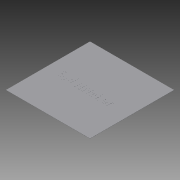
# Autodesk Inventor part: test
Saved by Autodesk Inventor 2015 SP1 (Build 190203100, 203)
## iProperties
Created: 2015-01-20
Part Number: test
Material: Generic
Document SubType Name: Modeling
Designer: Patrick
Density: 1 g/cm^3
Appearance: Default
Author: Patrick
Autodesk Inventor part; units mm, degrees
ref_plane "YZ Plane" through (0, 0, 0) normal (1, 0, 0) x (0, 1, 0)
ref_plane "XZ Plane" through (0, 0, 0) normal (0, 1, 0) x (-1, 0, 0)
ref_plane "XY Plane" through (0, 0, 0) normal (0, 0, 1) x (1, 0, 0)
sketch "Sketch1" plane through (0, 0, 0) normal (0, 0, 1) x (1, 0, 0)
  line L0 (-2500, 2500) -> (2500, 2500)
  line L1 (2500, 2500) -> (2500, -2500)
  line L2 (2500, -2500) -> (-2500, -2500)
  line L3 (-2500, -2500) -> (-2500, 2500)
  line L4 (-2500, 2500) -> (2500, -2500) construction
  line L5 (2500, 2500) -> (-2500, -2500) construction
  point P0 (0, 0)
  dimension "d0" = 5000
  dimension "d1" = 5000
  constraints: 12 end point, 2 midpoint, 2 parallel, 1 horizontal, 1 perpendicular
  measures "d0" distance of L1.end L2.end
  measures "d1" distance of L0.end L1.end
extrude "Extrusion1" add sketch "Sketch1" along normal blind 10
sketch "Sketch2" plane through (0, 0, 10) normal (0, 0, 1) x (1, 0, 0)
  spline S0 degree 4 poles (-1762.1962, 1575.4295) (-1491.5954, 1596.7242) (-1645.2682, 1599.4427) (-955.1929, 1604.26) (-825.0031, 1592.0214) (-732.519, 1582.853) (-459.1878, 1545.7413) (-345.6079, 1530.4798) (-181.1613, 1505.3471) (-45.0314, 1482.7736) (33.2926, 1462.2915) (239.3471, 1405.6013) (464.1859, 1340.1213) (686.0681, 1238.9414) (872.8585, 1134.1355) (1059.3908, 984.8503) (1135.6727, 916.3268) (1228.891, 830.1566) (1303.68, 755.6016) (1398.7078, 654.9396) (1484.4134, 536.3515) (1554.6482, 423.2358) (1622.964, 278.6899) (1656.5725, 195.5181) (1688.0679, 109.6167) (1711.1354, 34.6912) (1726.7352, -56.2271) (1732.0908, -96.9036) (1745.8175, -221.0892) (1754.6807, -282.6204) (1757.8584, -312.0265) (1759.1649, -327.9955) (1751.7151, -450.1044) (1749.3478, -483.8897) (1742.4101, -550.3074) (1733.7713, -624.2147) (1724.9155, -692.4119) (1713.0594, -760.8257) (1693.9812, -834.1715) (1666.2811, -923.9302) (1643.7916, -992.4869) (1601.981, -1107.4142) (1598.9852, -1125.3949) (1552.4445, -1217.5749) (1546.4569, -1240.9001) (1522.3305, -1296.4362) (1488.9966, -1328.7325) (1439.4405, -1364.0425) (1390.8946, -1389.0179) (1235.7237, -1476.0426) (1078.0613, -1526.58) (1029.0921, -1562.0631) (774.2297, -1615.128) (793.6908, -1622.9048) (755.7069, -1618.0314) (746.9426, -1630.276) (794.5654, -1458.788) (838.2853, -1308.0396) (850.1486, -1200.7586) (788.6595, -1247.2043) (738.5107, -1232.948) (505.6315, -1319.0728) (371.9051, -1351.4552) (170.8434, -1425.6846) (0.3667, -1497.8904) (-158.3591, -1567.0933) (-305.4965, -1632.8743) (-464.732, -1704.8026) (-562.0019, -1750.703) (-667.0386, -1801.7065) (-771.6429, -1855.0863) (-855.1097, -1895.1947) (-942.1183, -1946.1312) (-1006.5826, -1969.258) (-1131.0376, -2063.8301) (-1044.5072, -1892.2007) (-1066.3114, -1908.4549) (-1003.7573, -1699.41) (-977.9555, -1570.6674) (-934.5888, -1396.7403) (-900.0619, -1241.8358) (-878.6191, -1126.4711) (-860.2727, -1014.4476) (-841.1424, -887.8249) (-829.3125, -810.2865) (-819.1465, -727.3894) (-810.8924, -648.5496) (-803.9347, -562.191) (-795.8323, -453.4885) (-789.5667, -352.3094) (-784.6857, -245.5127) (-781.7139, -146.1831) (-779.9272, -44.8844) (-781.2254, 55.4386) (-787.9793, 179.1486) (-811.3684, 376.6004) (-842.439, 538.5854) (-892.2084, 725.6609) (-936.4315, 857.2935) (-978.7899, 950.9207) (-1037.4119, 1054.4206) (-1088.0468, 1135.0533) (-1275.6307, 1378.281) (-1438.3377, 1466.0297) (-1614.8909, 1557.3421) (-1762.1962, 1575.4295) knots 0 0 0 0 0 0.034839 0.046927 0.059157 0.069708 0.081008 0.092632 0.102748 0.113022 0.124139 0.136453 0.150242 0.164315 0.177048 0.188474 0.198679 0.20821 0.218183 0.228603 0.239498 0.249955 0.2597 0.268704 0.276906 0.284701 0.293012 0.300958 0.30789 0.314001 0.319872 0.325799 0.332476 0.340159 0.347396 0.354762 0.362372 0.370178 0.378285 0.38679 0.394808 0.402697 0.409774 0.416193 0.422676 0.428714 0.435047 0.442657 0.451726 0.462242 0.473798 0.483006 0.490066 0.494813 0.499083 0.50655 0.514493 0.522901 0.530604 0.537808 0.54693 0.558108 0.570873 0.583364 0.595556 0.607419 0.618543 0.629115 0.639153 0.64851 0.657648 0.666651 0.67507 0.683395 0.690966 0.698954 0.708235 0.71845 0.730094 0.741477 0.752176 0.762313 0.771652 0.780544 0.78896 0.796972 0.80531 0.814025 0.823107 0.832341 0.841416 0.850322 0.859373 0.869335 0.880255 0.892159 0.904186 0.91528 0.925458 0.934737 0.944559 0.95535 0.967093 1 1 1 1 1
  spline S1 degree 3 poles (809.627, -1569.6922) (882.146, -1551.6939) (955.9648, -1539.7281) (1025.1004, -1514.7845) (1138.5967, -1473.8468) (1251.7259, -1429.4464) (1342.7492, -1345.1899) (1381.8811, -1308.975) (1386.3757, -1249.1759) (1322.7566, -1223.4286) (1264.9716, -1200.0626) (1228.2905, -1195.0521) (1143.7263, -1201.3922) (1059.1523, -1207.7322) (987.8338, -1206.8988) (893.0005, -1228.9154) (866.6877, -1326.5963) (832.7748, -1465.8498) (809.627, -1569.6922) knots 0 0 0 0 1 1 1 2 2 2 3 3 3 4 4 4 5 5 5 6 6 6 6
  line L0 (-1821.1799, -36.4172) -> (-1734.2301, -27.9919)
  spline S2 degree 2 poles (-1734.2301, -27.9919) (-1726.4787, -71.8038) (-1678.2856, -112.9195) (-1637.8439, -112.9195) knots 0 0 0 1 2 2 2
  spline S3 degree 2 poles (-1637.8439, -112.9195) (-1594.706, -112.9195) (-1550.8941, -76.522) (-1550.8941, -51.9199) knots 0 0 0 1 2 2 2
  spline S4 degree 2 poles (-1550.8941, -51.9199) (-1550.8941, -36.0802) (-1569.4299, -14.1743) (-1592.3469, -6.0859) knots 0 0 0 1 2 2 2
  spline S5 degree 2 poles (-1592.3469, -6.0859) (-1607.8496, -0.6937) (-1663.794, 13.1239) knots 0 0 0 1 1 1
  spline S6 degree 2 poles (-1663.794, 13.1239) (-1735.5781, 30.9857) (-1764.5614, 56.9358) knots 0 0 0 1 1 1
  spline S7 degree 2 poles (-1764.5614, 56.9358) (-1805.3402, 93.3334) (-1805.3402, 145.5707) knots 0 0 0 1 1 1
  spline S8 degree 2 poles (-1805.3402, 145.5707) (-1805.3402, 179.6092) (-1766.9205, 238.2497) (-1694.7994, 268.918) (-1643.9102, 268.918) knots 0 0 0 1 2 3 3 3
  spline S9 degree 2 poles (-1643.9102, 268.918) (-1560.6675, 268.918) (-1476.4139, 196.1229) (-1474.3918, 135.1232) knots 0 0 0 1 2 2 2
  line L1 (-1474.3918, 135.1232) -> (-1563.7007, 131.079)
  spline S10 degree 2 poles (-1563.7007, 131.079) (-1569.4299, 165.1175) (-1607.1756, 195.1118) (-1644.9212, 195.1118) knots 0 0 0 1 2 2 2
  spline S11 degree 2 poles (-1644.9212, 195.1118) (-1684.0149, 195.1118) (-1705.9208, 179.2721) knots 0 0 0 1 1 1
  spline S12 degree 2 poles (-1705.9208, 179.2721) (-1720.0755, 168.8247) (-1720.0755, 151.6369) knots 0 0 0 1 1 1
  spline S13 degree 2 poles (-1720.0755, 151.6369) (-1720.0755, 136.1343) (-1706.9319, 124.6758) knots 0 0 0 1 1 1
  spline S14 degree 2 poles (-1706.9319, 124.6758) (-1689.7441, 110.5212) (-1559.3195, 79.8528) (-1496.9718, 47.1624) (-1461.5852, -9.7931) (-1461.5852, -51.9199) knots 0 0 0 1 2 3 4 4 4
  spline S15 degree 2 poles (-1461.5852, -51.9199) (-1461.5852, -89.6655) (-1503.7121, -156.0574) (-1580.8884, -188.4108) (-1638.5179, -188.4108) knots 0 0 0 1 2 3 3 3
  spline S16 degree 2 poles (-1638.5179, -188.4108) (-1722.4346, -188.4108) (-1812.4175, -110.8975) (-1821.1799, -36.4172) knots 0 0 0 1 2 2 2
  line L2 (-1389.4641, 139.8414) -> (-1310.2657, 139.8414)
  line L3 (-1310.2657, 139.8414) -> (-1310.2657, 92.6594)
  spline S17 degree 2 poles (-1310.2657, 92.6594) (-1294.763, 116.9244) (-1242.5257, 146.9187) (-1210.5093, 146.9187) knots 0 0 0 1 2 2 2
  spline S18 degree 2 poles (-1210.5093, 146.9187) (-1154.5649, 146.9187) (-1076.7145, 59.6319) (-1076.7145, -18.5555) knots 0 0 0 1 2 2 2
  spline S19 degree 2 poles (-1076.7145, -18.5555) (-1076.7145, -98.7649) (-1155.2389, -187.7368) (-1210.8463, -187.7368) knots 0 0 0 1 2 2 2
  spline S20 degree 2 poles (-1210.8463, -187.7368) (-1237.4705, -187.7368) (-1280.6084, -166.5049) (-1304.5364, -140.8918) knots 0 0 0 1 2 2 2
  line L4 (-1304.5364, -140.8918) -> (-1304.5364, -302.6588)
  line L5 (-1304.5364, -302.6588) -> (-1389.4641, -302.6588)
  line L6 (-1389.4641, -302.6588) -> (-1389.4641, 139.8414)
  spline S21 degree 2 poles (-1305.8845, -14.8483) (-1305.8845, -68.7706) (-1262.7466, -120.3339) (-1232.0783, -120.3339) knots 0 0 0 1 2 2 2
  spline S22 degree 2 poles (-1232.0783, -120.3339) (-1202.421, -120.3339) (-1162.9903, -73.1518) (-1162.9903, -19.2295) knots 0 0 0 1 2 2 2
  spline S23 degree 2 poles (-1162.9903, -19.2295) (-1162.9903, 30.9857) (-1203.432, 79.8528) (-1233.4263, 79.8528) knots 0 0 0 1 2 2 2
  spline S24 degree 2 poles (-1233.4263, 79.8528) (-1264.7687, 79.8528) (-1305.8845, 31.9967) (-1305.8845, -14.8483) knots 0 0 0 1 2 2 2
  line L7 (-1009.3116, -180.6595) -> (-1009.3116, 139.8414)
  line L8 (-1009.3116, 139.8414) -> (-924.3839, 139.8414)
  line L9 (-924.3839, 139.8414) -> (-924.3839, -180.6595)
  line L10 (-924.3839, -180.6595) -> (-1009.3116, -180.6595)
  line L11 (-1009.3116, 182.9793) -> (-1009.3116, 261.5037)
  line L12 (-1009.3116, 261.5037) -> (-924.3839, 261.5037)
  line L13 (-924.3839, 261.5037) -> (-924.3839, 182.9793)
  line L14 (-924.3839, 182.9793) -> (-1009.3116, 182.9793)
  line L15 (-690.1488, -295.5815) -> (-690.1488, 146.5817)
  line L16 (-690.1488, 146.5817) -> (-603.5361, 146.5817)
  line L17 (-603.5361, 146.5817) -> (-421.8852, -149.9912)
  line L18 (-421.8852, -149.9912) -> (-421.8852, 146.5817)
  line L19 (-421.8852, 146.5817) -> (-339.3166, 146.5817)
  line L20 (-339.3166, 146.5817) -> (-339.3166, -295.5815)
  line L21 (-339.3166, -295.5815) -> (-428.6255, -295.5815)
  line L22 (-428.6255, -295.5815) -> (-607.5802, -5.4119)
  line L23 (-607.5802, -5.4119) -> (-607.5802, -295.5815)
  line L24 (-607.5802, -295.5815) -> (-690.1488, -295.5815)
  line L25 (-243.9415, -295.5815) -> (-243.9415, 146.5817)
  line L26 (-243.9415, 146.5817) -> (-157.3287, 146.5817)
  line L27 (-157.3287, 146.5817) -> (24.3222, -149.9912)
  line L28 (24.3222, -149.9912) -> (24.3222, 146.5817)
  line L29 (24.3222, 146.5817) -> (106.8908, 146.5817)
  line L30 (106.8908, 146.5817) -> (106.8908, -295.5815)
  line L31 (106.8908, -295.5815) -> (17.5819, -295.5815)
  line L32 (17.5819, -295.5815) -> (-161.3729, -5.4119)
  line L33 (-161.3729, -5.4119) -> (-161.3729, -295.5815)
  line L34 (-161.3729, -295.5815) -> (-243.9415, -295.5815)
  line L35 (263.9396, -72.8148) -> (187.1003, -58.9972)
  spline S25 degree 2 poles (187.1003, -58.9972) (200.2438, -12.4892) (263.6026, 31.9967) (325.9503, 31.9967) knots 0 0 0 1 2 2 2
  spline S26 degree 2 poles (325.9503, 31.9967) (382.9058, 31.9967) (438.5132, 5.0356) (461.0932, -36.0802) (461.0932, -91.3506) knots 0 0 0 1 2 3 3 3
  line L36 (461.0932, -91.3506) -> (459.7451, -190.4329)
  spline S27 degree 2 poles (459.7451, -190.4329) (459.7451, -232.5597) (467.8335, -272.6645) (478.9549, -295.5815) knots 0 0 0 1 2 2 2
  line L37 (478.9549, -295.5815) -> (395.0383, -295.5815)
  spline S28 degree 2 poles (395.0383, -295.5815) (391.6682, -287.1561) (386.9499, -270.6424) knots 0 0 0 1 1 1
  spline S29 degree 2 poles (386.9499, -270.6424) (384.9279, -262.8911) (383.9168, -260.532) knots 0 0 0 1 1 1
  spline S30 degree 2 poles (383.9168, -260.532) (362.3479, -281.4269) (312.8067, -302.6588) (284.8345, -302.6588) knots 0 0 0 1 2 2 2
  spline S31 degree 2 poles (284.8345, -302.6588) (235.2934, -302.6588) (178.3379, -249.0735) (178.3379, -207.9577) knots 0 0 0 1 2 2 2
  spline S32 degree 2 poles (178.3379, -207.9577) (178.3379, -180.6595) (204.288, -138.1957) (251.133, -115.6157) (295.282, -107.1903) knots 0 0 0 1 2 3 3 3
  spline S33 degree 2 poles (295.282, -107.1903) (354.5965, -96.0688) (377.5135, -86.2954) knots 0 0 0 1 1 1
  line L38 (377.5135, -86.2954) -> (377.5135, -77.87)
  spline S34 degree 2 poles (377.5135, -77.87) (377.5135, -53.605) (353.2485, -32.7101) (319.884, -32.7101) knots 0 0 0 1 2 2 2
  spline S35 degree 2 poles (319.884, -32.7101) (297.3041, -32.7101) (271.6909, -50.5718) (263.9396, -72.8148) knots 0 0 0 1 2 2 2
  spline S36 degree 2 poles (377.5135, -141.5658) (361.3368, -146.958) (290.5638, -162.1237) (279.7793, -169.201) knots 0 0 0 1 2 2 2
  spline S37 degree 2 poles (279.7793, -169.201) (263.2656, -180.9965) (263.2656, -199.1953) knots 0 0 0 1 1 1
  spline S38 degree 2 poles (263.2656, -199.1953) (263.2656, -217.0571) (289.8897, -243.0072) (310.4476, -243.0072) knots 0 0 0 1 2 2 2
  spline S39 degree 2 poles (310.4476, -243.0072) (333.3646, -243.0072) (353.9225, -227.8415) knots 0 0 0 1 1 1
  spline S40 degree 2 poles (353.9225, -227.8415) (369.4252, -216.383) (374.1434, -199.8693) knots 0 0 0 1 1 1
  spline S41 degree 2 poles (374.1434, -199.8693) (377.5135, -189.0849) (377.5135, -158.4165) knots 0 0 0 1 1 1
  line L39 (377.5135, -158.4165) -> (377.5135, -141.5658)
  line L40 (541.3026, -295.5815) -> (541.3026, 146.5817)
  line L41 (541.3026, 146.5817) -> (626.2303, 146.5817)
  line L42 (626.2303, 146.5817) -> (626.2303, -87.9805)
  line L43 (626.2303, -87.9805) -> (725.3126, 24.9194)
  line L44 (725.3126, 24.9194) -> (829.7872, 24.9194)
  line L45 (829.7872, 24.9194) -> (720.2574, -92.3617)
  line L46 (720.2574, -92.3617) -> (837.5385, -295.5815)
  line L47 (837.5385, -295.5815) -> (746.2075, -295.5815)
  line L48 (746.2075, -295.5815) -> (665.324, -151.6762)
  line L49 (665.324, -151.6762) -> (626.2303, -193.129)
  line L50 (626.2303, -193.129) -> (626.2303, -295.5815)
  line L51 (626.2303, -295.5815) -> (541.3026, -295.5815)
  line L52 (1073.1117, -193.4661) -> (1157.7024, -207.6207)
  spline S42 degree 2 poles (1157.7024, -207.6207) (1141.5257, -254.1287) (1071.0897, -302.6588) (1018.1784, -302.6588) knots 0 0 0 1 2 2 2
  spline S43 degree 2 poles (1018.1784, -302.6588) (934.5987, -302.6588) (894.494, -248.0624) knots 0 0 0 1 1 1
  spline S44 degree 2 poles (894.494, -248.0624) (862.8146, -204.2505) (862.8146, -137.8586) knots 0 0 0 1 1 1
  spline S45 degree 2 poles (862.8146, -137.8586) (862.8146, -57.9862) (946.0572, 31.9967) (1009.753, 31.9967) knots 0 0 0 1 2 2 2
  spline S46 degree 2 poles (1009.753, 31.9967) (1081.2001, 31.9967) (1163.7687, -62.3674) (1162.0836, -159.7646) knots 0 0 0 1 2 2 2
  line L53 (1162.0836, -159.7646) -> (949.7644, -159.7646)
  spline S47 degree 2 poles (949.7644, -159.7646) (950.7754, -197.5102) (989.8691, -239.3) (1019.1894, -239.3) knots 0 0 0 1 2 2 2
  spline S48 degree 2 poles (1019.1894, -239.3) (1039.0733, -239.3) (1066.0344, -217.7311) (1073.1117, -193.4661) knots 0 0 0 1 2 2 2
  spline S49 degree 2 poles (1077.8299, -107.8643) (1076.8189, -71.1297) (1040.7583, -32.7101) (1014.8082, -32.7101) knots 0 0 0 1 2 2 2
  spline S50 degree 2 poles (1014.8082, -32.7101) (987.173, -32.7101) (968.9742, -52.9309) knots 0 0 0 1 1 1
  spline S51 degree 2 poles (968.9742, -52.9309) (951.1124, -73.1518) (951.1124, -107.8643) knots 0 0 0 1 1 1
  line L54 (951.1124, -107.8643) -> (1077.8299, -107.8643)
  line L55 (1312.3921, -295.5815) -> (1227.4644, -295.5815)
  line L56 (1227.4644, -295.5815) -> (1227.4644, 24.9194)
  line L57 (1227.4644, 24.9194) -> (1306.3259, 24.9194)
  line L58 (1306.3259, 24.9194) -> (1306.3259, -20.5775)
  spline S52 degree 2 poles (1306.3259, -20.5775) (1326.5467, 11.7759) (1358.5631, 31.9967) (1379.121, 31.9967) knots 0 0 0 1 2 2 2
  spline S53 degree 2 poles (1379.121, 31.9967) (1408.1043, 31.9967) (1434.7284, 15.82) knots 0 0 0 1 1 1
  line L59 (1434.7284, 15.82) -> (1408.7783, -57.9862)
  spline S54 degree 2 poles (1408.7783, -57.9862) (1387.2094, -44.1686) (1369.0106, -44.1686) knots 0 0 0 1 1 1
  spline S55 degree 2 poles (1369.0106, -44.1686) (1351.1488, -44.1686) (1326.5467, -63.7154) (1312.3921, -114.9416) (1312.3921, -196.8362) knots 0 0 0 1 2 3 3 3
  line L60 (1312.3921, -196.8362) -> (1312.3921, -295.5815)
  point P0 (0, 0)
  point P1 (-1843.4228, -302.6588)
  point P2 (-735.9828, -302.6588)
  point P3 (-1305.4717, 1600.2698)
  point P4 (-901.4043, 1596.6678)
  point P5 (-817.2551, 1591.0616)
  point P6 (-730.557, 1581.5134)
  point P7 (-481.5639, 1548.7979)
  point P8 (-323.6048, 1526.7522)
  point P9 (-168.7972, 1502.9543)
  point P10 (-54.2816, 1482.7334)
  point P11 (26.8797, 1463.5477)
  point P12 (198.2917, 1416.4538)
  point P13 (450.7979, 1337.2988)
  point P14 (688.5922, 1232.8753)
  point P15 (900.1451, 1105.9644)
  point P16 (1068.1441, 975.1309)
  point P17 (1147.7057, 904.8558)
  point P18 (1225.1076, 832.5743)
  point P19 (1299.938, 758.3326)
  point P20 (1390.4194, 658.9084)
  point P21 (1480.475, 538.3689)
  point P22 (1558.3356, 409.0303)
  point P23 (1624.8428, 270.8875)
  point P24 (1659.9862, 184.8494)
  point P25 (1687.9818, 106.9626)
  point P26 (1710.1321, 29.3546)
  point P27 (1724.7418, -46.8984)
  point P28 (1733.0303, -107.6059)
  point P29 (1748.3478, -236.5966)
  point P30 (1755.3451, -290.2769)
  point P31 (1757.3763, -308.5877)
  point P32 (1758.1112, -325.9923)
  point P33 (1752.7122, -432.5084)
  point P34 (1748.4279, -490.1866)
  point P35 (1742.4575, -548.221)
  point P36 (1733.7827, -622.5459)
  point P37 (1724.4388, -691.4626)
  point P38 (1712.537, -757.3807)
  point P39 (1694.0203, -831.1116)
  point P40 (1667.8031, -918.0696)
  point P41 (1638.1378, -1006.8416)
  point P42 (1605.4849, -1100.494)
  point P43 (1590.1092, -1140.5632)
  point P44 (1556.3308, -1213.2722)
  point P45 (1542.7956, -1247.4028)
  point P46 (1520.7268, -1291.5318)
  point P47 (1489.3835, -1326.2971)
  point P48 (1450.3126, -1355.1736)
  point P49 (1403.5203, -1382.7398)
  point P50 (1259.9422, -1457.1606)
  point P51 (1095.662, -1525.4064)
  point P52 (924.7292, -1582.0505)
  point P53 (785.9121, -1620.1151)
  point P54 (780.8451, -1620.8102)
  point P55 (766.6665, -1620.5509)
  point P56 (756.9477, -1620.2198)
  point P57 (776.569, -1524.6638)
  point P58 (839.9217, -1259.9255)
  point P59 (829.8692, -1226.8004)
  point P60 (803.4115, -1231.8832)
  point P61 (759.0566, -1241.6347)
  point P62 (562.6543, -1296.1178)
  point P63 (364.0532, -1358.2165)
  point P64 (170.342, -1428.0065)
  point P65 (-5.7616, -1500.97)
  point P66 (-161.9914, -1569.0509)
  point P67 (-318.5867, -1638.9141)
  point P68 (-469.7263, -1707.621)
  point P69 (-569.7772, -1754.7258)
  point P70 (-670.6374, -1804.0161)
  point P71 (-773.2892, -1855.3798)
  point P72 (-859.7442, -1899.4376)
  point P73 (-940.3171, -1941.9605)
  point P74 (-1028.3033, -1989.1065)
  point P75 (-1090.034, -2011.9951)
  point P76 (-1064.6967, -1926.7065)
  point P77 (-1054.5893, -1889.8503)
  point P78 (-1021.1755, -1753.3945)
  point P79 (-975.5568, -1566.4805)
  point P80 (-933.1134, -1386.6193)
  point P81 (-899.2462, -1232.8176)
  point P82 (-878.1128, -1120.5347)
  point P83 (-859.0962, -1004.9756)
  point P84 (-840.4542, -883.372)
  point P85 (-828.842, -803.2622)
  point P86 (-819.5419, -728.2397)
  point P87 (-811.7069, -652.9392)
  point P88 (-804.42, -566.7822)
  point P89 (-796.4212, -458.0443)
  point P90 (-789.8243, -350.508)
  point P91 (-784.9621, -243.8992)
  point P92 (-781.9289, -144.3915)
  point P93 (-780.5675, -49.6465)
  point P94 (-781.7833, 43.0345)
  point P95 (-788.6718, 163.3228)
  point P96 (-811.4848, 358.8917)
  point P97 (-848.2175, 551.5643)
  point P98 (-899.1815, 741.0826)
  point P99 (-942.7525, 866.5971)
  point P100 (-983.2412, 955.2453)
  point P101 (-1030.9414, 1041.4981)
  point P102 (-1084.8994, 1125.7712)
  point P103 (-1206.4005, 1277.6166)
  point P104 (-1358.7884, 1409.3168)
  point P105 (-1533.7075, 1507.4688)
  point P106 (943.0747, -1539.0153)
  point P107 (984.0181, -1528.0801)
  point P108 (1023.8566, -1515.2317)
  point P109 (1091.9365, -1489.9211)
  point P110 (1156.9612, -1462.9125)
  point P111 (1188.1535, -1448.3039)
  point P112 (1218.4323, -1432.7085)
  point P113 (1247.7559, -1415.9521)
  point P114 (1276.0776, -1397.8657)
  point P115 (1303.3501, -1378.28)
  point P116 (1329.4562, -1357.0819)
  point P117 (1346.707, -1341.3262)
  point P118 (1354.8361, -1331.8324)
  point P119 (1361.4356, -1321.7524)
  point P120 (1366.4274, -1311.2907)
  point P121 (1369.7499, -1300.6401)
  point P122 (1371.3543, -1289.9743)
  point P123 (1371.1967, -1279.4429)
  point P124 (1369.2237, -1269.1699)
  point P125 (1365.355, -1259.2607)
  point P126 (1359.4684, -1249.8154)
  point P127 (1351.3891, -1240.9469)
  point P128 (1340.8885, -1232.7982)
  point P129 (1327.4507, -1225.4453)
  point P130 (1311.5637, -1219.0372)
  point P131 (1283.1331, -1209.475)
  point P132 (1256.161, -1203.2097)
  point P133 (1227.6712, -1199.7522)
  point P134 (1194.5806, -1198.9129)
  point P135 (1153.2906, -1200.7103)
  point P136 (1053.0701, -1207.0275)
  point P137 (1005.9244, -1210.7331)
  point P138 (958.4128, -1216.4947)
  point P139 (908.1537, -1225.546)
  point P140 (894.3014, -1228.6145)
  point P141 (889.236, -1242.9785)
  point P142 (880.5873, -1275.8854)
  point P143 (843.4751, -1424.3826)
  point P144 (-1762.1438, 1574.7634)
  constraints: 149 other
emboss "Emboss1" sketch "Sketch2" operation add depth 5 direction (0, 0, -1) contours L0 S2 S3 S4 S5 S6 S7 S8 S9 L1 S10 S11 S12 S13 S14 S15 S16 | L2 L3 S17 S18 S19 S20 L4 L5 L6 | L7 L8 L9 L10 | L11 L12 L13 L14 | L15 L16 L17 L18 L19 L20 L21 L22 L23 L24 | L25 L26 L27 L28 L29 L30 L31 L32 L33 L34 | L35 S25 S26 L36 S27 L37 S28 S29 S30 S31 S32 S33 L38 S34 S35 | L40 L41 L42 L43 L44 L45 L46 L47 L48 L49 L50 L51 | L52 S42 S43 S44 S45 S46 L53 S47 S48 | L55 L56 L57 L58 S52 S53 L59 S54 S55 L60
body "Solid1"
